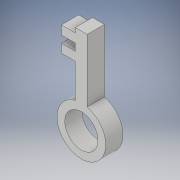
# Autodesk Inventor part: Key
Saved by Autodesk Inventor 2017 (Build 210142000, 142)
## iProperties
Created: 2019-05-01
Part Number: Key
Material: Generic
Document SubType Name: Modeling
Designer: Jessica
Density: 1 g/cm^3
Appearance: Default
Author: Jessica
Autodesk Inventor part; units mm, degrees
ref_plane "YZ Plane" through (0, 0, 0) normal (1, 0, 0) x (0, 1, 0)
ref_plane "XZ Plane" through (0, 0, 0) normal (0, 1, 0) x (-1, 0, 0)
ref_plane "XY Plane" through (0, 0, 0) normal (0, 0, 1) x (1, 0, 0)
sketch "Sketch1" plane through (0, 0, 0) normal (0, 0, 1) x (1, 0, 0)
  arc A0 (-2.6945, 10.3961) -> (2.5563, 10.431) centre (0, 0) ccw
  circle A1 centre (0, 0) radius 7.3439
  line L0 (-2.6945, 38.1942) -> (2.5563, 38.1942)
  line L1 (-8.8208, 36.1476) -> (-2.6945, 36.1476)
  line L2 (-2.6945, 32.2644) -> (-8.8208, 32.2644)
  line L3 (-8.8208, 32.2644) -> (-8.8208, 36.1476)
  line L4 (-8.8208, 29.1799) -> (-2.6945, 29.1799)
  line L5 (-2.6945, 25.2966) -> (-8.8208, 25.2966)
  line L6 (-8.8208, 25.2966) -> (-8.8208, 29.1799)
  line L7 (-2.6945, 36.1476) -> (-2.6945, 38.1942)
  line L8 (-2.6945, 29.1799) -> (-2.6945, 32.2644)
  line L9 (-2.6945, 10.3961) -> (-2.6945, 25.2966)
  line L10 (2.5563, 38.1942) -> (2.5563, 10.431)
  constraints: 22 end point, 5 parallel, 3 horizontal, 2 centre point, 2 coincident, 2 point on circle, 1 perpendicular
extrude "Extrusion1" add sketch "Sketch1" along normal blind 7.62
body "Solid1"
